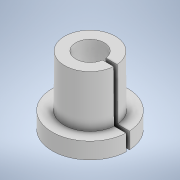
# Autodesk Inventor part: くさび
Saved by Autodesk Inventor 2020 (Build 240168000, 168)
## iProperties
Created: 2019-10-29
Part Number: くさび
Material: 一般
Document SubType Name: Modeling
Designer: highs
Density: 1 g/cm^3
Appearance: 既定
Author: highs
## iProperties of the stored document _3D プリント.ipt
Created: 2019-10-29
Part Number: _3D プリント
Material: 一般
Document SubType Name: Modeling
Designer: highs
Density: 1 g/cm^3
Appearance: 既定
Author: highs
Autodesk Inventor part; units mm, degrees
ref_plane "YZ Plane" through (0, 0, 0) normal (1, 0, 0) x (0, 1, 0)
ref_plane "XZ Plane" through (0, 0, 0) normal (0, 1, 0) x (-1, 0, 0)
ref_plane "XY Plane" through (0, 0, 0) normal (0, 0, 1) x (1, 0, 0)
sketch "スケッチ1" plane through (0, 0, 0) normal (0, 0, 1) x (1, 0, 0)
  line L0 (0, 0) -> (8.3, 0) construction
  line L1 (8.3, 0) -> (8.3, 39.5)
  line L2 (8.3, 39.5) -> (0, 39.5) construction
  line L3 (0, 39.5) -> (0, 0) construction
  line L4 (8.3, 39.5) -> (14.8, 39.5)
  line L5 (14.8, 39.5) -> (15.05, 9.5)
  line L6 (15.05, 9.5) -> (22, 9.5)
  line L7 (22, 9.5) -> (22, 0)
  line L8 (22, 0) -> (8.3, 0)
  dimension "d0" = 8.3
  dimension "d1" = 30
  dimension "d2" = 9.5
  dimension "d3" = 0.25
  dimension "d4" = 15.05
  dimension "d5" = 22
  dimension "d12" = 14.8
  constraints: 18 end point, 3 horizontal, 3 perpendicular, 2 parallel
  measures "d0" distance of L0.start L0.end
  measures "d1" distance between parallel lines of L4 L6
  measures "d2" distance of L6.end L7.end
  measures "d3" horizontal distance of L4.end L5.end
  measures "d4" distance from line of L3 L5.end
  measures "d5" distance between parallel lines of L3 L7
  measures "d12" distance from line of L3 L4.end
revolve "回転1" add sketch "スケッチ1" angle 360 about axis through (0, 39.5, 0) along (0, -1, 0)
sketch "スケッチ2" plane through (0, 0, 0) normal (0, -1, 0) x (1, 0, 0)
  line L0 (0, 0) -> (35, 0) construction
  line L1 (5, -1) -> (30, -1)
  line L2 (30, -1) -> (30, 1)
  line L3 (30, 1) -> (5, 1)
  line L4 (5, 1) -> (5, -1)
  line L5 (5, -1) -> (30, 1) construction
  line L6 (30, -1) -> (5, 1) construction
  point P0 (17.5, 0)
  dimension "d7" = 2
  dimension "d8" = 30
  dimension "d9" = 5
  constraints: 14 end point, 3 midpoint, 2 horizontal, 2 parallel, 1 perpendicular
  measures "d7" distance of L1.end L2.end
  measures "d8" distance from line of L2 L0.start
  measures "d9" distance from line of L0.start L4
extrude "押し出し1" cut sketch "スケッチ2" against normal through all
